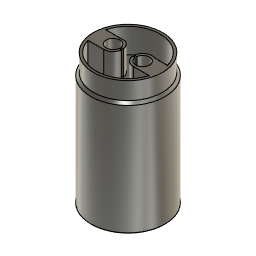
Bottom fan tube (temp sensor holders) (Autodesk Fusion 360 design; units mm, degrees)
Autodesk Fusion 360 part; units mm, degrees
sketch "Sketch1" plane through (0, 0, 0) normal (0, 0, 1) x (1, 0, 0)
  circle A0 centre (0, 0) radius 13
  circle A1 centre (0, 0) radius 14
  circle A2 centre (0, 0) radius 6 construction
  line L0 (-18, -0.0439) -> (20, -0.0439) construction
  line L1 (0, 17) -> (0, -15) construction
  circle A3 centre (-5.9998, -0.0439) radius 2.8
  circle A4 centre (5.9998, -0.0439) radius 2.8
  circle A5 centre (5.9998, -0.0439) radius 3.8
  circle A6 centre (-5.9998, -0.0439) radius 3.8
  line L2 (-18, -0.0439) -> (-18, 3.4561) construction
  line L3 (-18, 3.4561) -> (29, 3.4561) construction
  line L4 (-25, -0.3439) -> (-25, -3.8439) construction
  line L5 (-25, -3.8439) -> (28, -3.8439) construction
  line L6 (-4.52, 3.4561) -> (-12.5322, 3.4561)
  line L7 (-12.4187, -3.8439) -> (-5.9998, -3.8439)
  line L8 (7.4797, 3.4561) -> (12.5322, 3.4561)
  line L9 (5.9998, -3.8439) -> (12.4187, -3.8439)
  line L10 (6.6591, -0.3553) -> (-6.6591, -0.3553)
  line L11 (-6.6591, -0.3553) -> (-6.6591, 0.3553)
  line L12 (-6.6591, 0.3553) -> (6.6591, 0.3553)
  line L13 (6.6591, 0.3553) -> (6.6591, -0.3553)
  line L14 (6.6591, -0.3553) -> (-6.6591, 0.3553) construction
  line L15 (-6.6591, -0.3553) -> (6.6591, 0.3553) construction
  dimension "d1" = 26
  dimension "d2" = 28
  dimension "d3" = 12
  dimension "d4" = 5.6
  dimension "d5" = 5.6
  dimension "d6" = 7.6
  dimension "d7" = 7.6
  dimension "d8" = 3.5
  dimension "d9" = 47
  dimension "d10" = 3.5
  dimension "d11" = 53
  dimension "d12" = 0.7105
  constraint coincident A0.centre A1.centre
  constraint concentric A0 A2
  constraint horizontal L0
  constraint vertical L1
  constraint coincident L0 A3.centre
  constraint coincident A2 A3.centre
  constraint coincident L0 A4.centre
  constraint coincident A2 A4.centre
  constraint concentric A4 A5
  constraint concentric A3 A6
  constraint perpendicular L0 L2
  constraint perpendicular L2 L3
  constraint vertical L4
  constraint perpendicular L4 L5
  constraint coincident L3 L6.start
  constraint coincident A6 L6.start
  constraint coincident L3 L6.end
  constraint coincident A0 L6.end
  constraint coincident L5 L7.start
  constraint coincident A0 L7.start
  constraint coincident A6 L7.end
  constraint coincident L5 L7.end
  constraint tangent A6 L7
  constraint coincident L3 L8.start
  constraint coincident A5 L8.start
  constraint coincident L3 L8.end
  constraint coincident A0 L8.end
  constraint coincident L5 L9.start
  constraint coincident A5 L9.start
  constraint coincident A0 L9.end
  constraint coincident L5 L9.end
  constraint horizontal L10
  constraint perpendicular L10 L11
  constraint parallel L10 L12
  constraint parallel L11 L13
  constraint coincident L14 A0.centre
  constraint coincident L15 A0.centre
  measures "d1" diameter of A0
  measures "d2" diameter of A1
  measures "d3" diameter of A2
  measures "d4" diameter of A3
  measures "d5" diameter of A4
  measures "d6" diameter of A5
  measures "d7" diameter of A6
  measures "d8" distance of L0.start L2.end
  measures "d9" distance of L2.end L3.end
  measures "d10" distance of L4.start L4.end
  measures "d11" distance of L4.end L5.end
  measures "d12" distance of L10.start L12.end
extrude "Extrude3" add sketch "Sketch1" along normal blind 10 contours A0 A5 L8 L9 | A0 A6 L6 L7 | A4 A5 L10 L12 | A3 A6 L6 L10 L12 | A1 picked at (2.5768, -0.5414) makes body 1
extrude "Extrude1" add sketch "Sketch1" along normal blind 4 separate body contours A0 A5 L8 L9 | A0 A6 L6 L7 | A4 A5 L10 L12 | A1 picked at (2.5768, -0.5414) makes body 2
ref_plane "WorkPlane1" through (0, 0, 2) normal (0, 0, -1) x (-1, 0, 0)
sketch "Sketch2" plane through (0, 0, 2) normal (0, 0, -1) x (1, 0, 0)
  circle A0 centre (0, 0) radius 15
  circle A1 centre (0, 0) radius 14
  dimension "d16" = 30
  dimension "d17" = 28
  constraint coincident A0.centre A1.centre
  measures "d16" diameter of A0
  measures "d17" diameter of A1
extrude "Extrude2" add sketch "Sketch2" along normal blind 45 bodies 2 1
fillet "Fillet1" radius 0.3 1 edges at (-13.9849, 5.4242, -43) on bodies 2
fillet "Fillet2" radius 0.3 1 edges at (-13.0526, -5.0626, -43) on bodies 2
chamfer "Chamfer1" distance 1 angle 45 1 edges at (-13.0526, -5.0626, 2) on bodies 2
